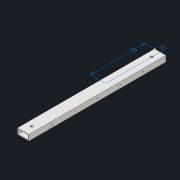
# Autodesk Inventor part: Back Bar
Saved by Autodesk Inventor 2022 (Build 260153000, 153)
## iProperties
Created: 2022-09-10
Part Number: Back Bar
Material: Generic
Document SubType Name: Modeling
Designer: robpl
Density: 1 g/cm^3
Appearance: Default
Author: robpl
Autodesk Inventor part; units mm, degrees
ref_plane "YZ Plane" through (0, 0, 0) normal (1, 0, 0) x (0, 1, 0)
ref_plane "XZ Plane" through (0, 0, 0) normal (0, 1, 0) x (-1, 0, 0)
ref_plane "XY Plane" through (0, 0, 0) normal (0, 0, 1) x (1, 0, 0)
sketch "Sketch1" plane through (0, 0, 0) normal (0, 0, 1) x (1, 0, 0)
  line L0 (0, 0) -> (50, 0)
  line L1 (50, 0) -> (50, 25)
  line L2 (50, 25) -> (0, 25)
  line L3 (0, 25) -> (0, 0)
  line L4 (47, 3) -> (3, 3)
  line L5 (3, 3) -> (3, 22)
  line L6 (3, 22) -> (47, 22)
  line L7 (47, 22) -> (47, 3)
  dimension "d0" = 50
  dimension "d1" = 25
  dimension "d2" = 3
  constraints: 16 end point, 4 parallel, 2 perpendicular, 1 horizontal, 3 other
  measures "d0" distance of L2.end L1.end
  measures "d1" distance of L1.end L0.end
  measures "d2" distance between parallel lines of L0 L4
extrude "Extrusion1" add sketch "Sketch1" along normal blind 600
sketch "Sketch2" plane through (0, 25, 0) normal (0, 1, 0) x (1, 0, 0)
  line L0 (50, -600) -> (0, -600) projected
  point P0 (0, 0)
  point P1 (25, -562.5)
  point P2 (25, -37.5)
  dimension "d5" = 37.5
  dimension "d6" = 37.5
  dimension "d7" = 25
  constraints: 1 vertical alignment
  measures "d5" vertical distance of point (0, 0) point (25, -37.5)
  measures "d6" distance from line of L0 point (25, -562.5)
  measures "d7" horizontal distance of point (0, 0) point (25, -37.5)
hole "Hole1" at (25, 25, 562.5) at (25, 25, 37.5) direction (0, -1, 0) diameter 6 end through all counterbore diameter 11 counterbore depth 5
sketch "Sketch4" plane through (50, 0, 0) normal (1, 0, 0) x (0, 0, -1)
  line L0 (0, 0) -> (66.9632, 0)
  point P0 (-100, 12.5)
  point P1 (-200, 12.5)
  point P2 (-300, 12.5)
  point P3 (-400, 12.5)
  point P4 (-500, 12.5)
  dimension "d31" = 100
  dimension "d32" = 12.5
  dimension "d36" = 100
  constraints: 2 end point, 2 horizontal, 4 other
  measures "d31" horizontal distance of L0.start point (-100, 12.5)
  measures "d32" vertical distance of L0.start point (-100, 12.5)
  measures "d36" distance of point (-100, 12.5) point (-200, 12.5)
hole "Hole3" at (50, 12.5, 100) at (50, 12.5, 200) at (50, 12.5, 300) at (50, 12.5, 400) at (50, 12.5, 500) direction (-1, 0, 0) diameter 5 depth 8 tip angle 118
sketch "Sketch6" plane through (0, 25, 0) normal (0, 1, 0) x (1, 0, 0)
  line L0 (50, -600) -> (0, -600) projected
  point P0 (0, 0)
  point P1 (29, -239)
  point P2 (29, -361)
  dimension "d60" = 239
  dimension "d61" = 29
  dimension "d69" = 239
  constraints: 1 vertical alignment
  measures "d60" vertical distance of point (0, 0) point (29, -239)
  measures "d61" horizontal distance of point (0, 0) point (29, -239)
  measures "d69" distance from line of L0 point (29, -361)
hole "Hole5" at (29, 25, 239) at (29, 25, 361) direction (0, -1, 0) diameter 28.575 end through all
sketch "Sketch7" plane through (0, 0, 0) normal (0, 1, 0) x (1, 0, 0)
  line L0 (50, 0) -> (50, -600) projected
  line L1 (50, 0) -> (0, 0) projected
  point P0 (41, -330)
  point P1 (9, -330)
  point P2 (9, -270)
  point P3 (41, -270)
  dimension "d70" = 9
  dimension "d71" = 9
  dimension "d72" = 60
  dimension "d73" = 600
  dimension "d74" = 270
  constraints: 2 horizontal alignment, 2 vertical alignment
  measures "d70" horizontal distance of L1.end point (9, -270)
  measures "d71" distance from line of L0 point (41, -270)
  measures "d72" distance of point (41, -330) point (41, -270)
  measures "d73" distance of L0.start L0.end
  measures "d74" distance from line of L1 point (41, -270)
hole "Hole6" at (41, 0, 330) at (9, 0, 330) at (9, 0, 270) at (41, 0, 270) direction (0, 1, 0) diameter 5 depth 8
equation "\"d69\" = d60"
equation "\"d71\" = d70"
body "Solid1"
